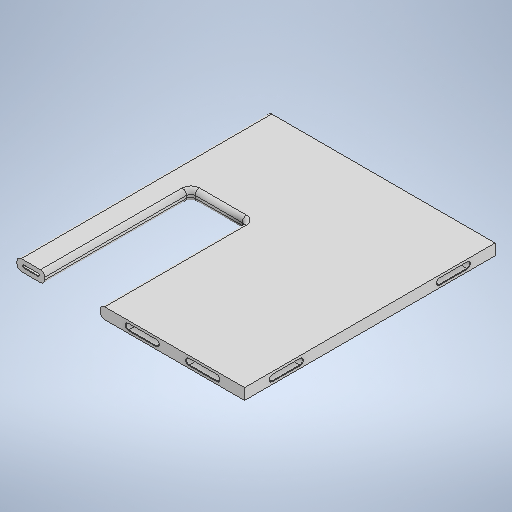
# Autodesk Inventor part: RightFlap4
Saved by Autodesk Inventor 2025.3 (Build 293356000, 356)
## iProperties
Created: 2025-11-19
Part Number: RightFlap4
Material: Generic
Document SubType Name: Modeling
Designer: User
Density: 1 g/cm^3
Appearance: Default
Author: User
Autodesk Inventor part; units mm, degrees
ref_plane "YZ Plane" through (0, 0, 0) normal (1, 0, 0) x (0, 1, 0)
ref_plane "XZ Plane" through (0, 0, 0) normal (0, 1, 0) x (-1, 0, 0)
ref_plane "XY Plane" through (0, 0, 0) normal (0, 0, 1) x (1, 0, 0)
sketch "Sketch1" plane through (0, 0, 0) normal (0, 1, 0) x (-1, 0, 0)
  line L0 (0, 0) -> (300, 0)
  line L1 (300, 0) -> (300, -420)
  line L2 (300, -420) -> (0, -420)
  line L3 (0, -420) -> (0, 0)
  line L4 (240, -150) -> (280, -150)
  line L5 (280, -150) -> (280, -270)
  line L6 (280, -270) -> (240, -270)
  line L7 (240, -270) -> (240, -150)
  line L8 (240, -150) -> (280, -270) construction
  line L9 (280, -150) -> (240, -270) construction
  dimension "d0" = 300
  dimension "d1" = 420
  dimension "d5" = 40
  dimension "d6" = 120
  constraints: 20 end point, 4 parallel, 2 horizontal, 2 perpendicular
  measures "d0" distance of L1.end L2.end
  measures "d1" distance of L0.end L1.end
  measures "d5" distance of L5.end L6.end
  measures "d6" distance of L4.end L5.end
extrude "Extrusion1" add sketch "Sketch1" along normal blind 8
sketch "Sketch2" plane through (0, 0, 0) normal (1, 0, 0) x (0, 0, -1)
  line L0 (150, 0) -> (270, 0) projected
  line L1 (210, 0) -> (210, 4)
  line L2 (420, 0) -> (420, 8) projected
  line L3 (0, 4.5) -> (420, 4.5)
  line L4 (420, 4.5) -> (420, 3.5)
  line L5 (420, 3.5) -> (0, 3.5)
  line L6 (0, 3.5) -> (0, 4.5)
  line L7 (0, 4.5) -> (420, 3.5) construction
  line L8 (420, 4.5) -> (0, 3.5) construction
  line L9 (0, 0) -> (0, 8) projected
  line L10 (420, 3.5) -> (0, 3.5)
  line L11 (0, 3.5) -> (0, 8)
  line L12 (0, 8) -> (420, 8)
  line L13 (420, 8) -> (420, 3.5)
  dimension "d7" = 4
  dimension "d8" = 1
  constraints: 22 end point, 4 parallel, 3 midpoint, 2 horizontal, 2 perpendicular, 1 point on line, 1 vertical
  measures "d7" distance of L1.start L1.end
  measures "d8" distance of L3.end L4.end
extrude "Extrusion2" cut sketch "Sketch2" against normal blind 40
fillet "Fillet1" radius 3.1 14 edges at (-300, 8, -210) (-300, 0, -210) (-280, 8, -210) (-260, 8, -270) (-240, 8, -210) (-280, 0, -210) (-260, 0, -270) (-280, 4, -270) (-240, 4, -270) (-240, 4, -150) (-260, 0, -150) (-260, 8, -150) (-280, 4, -150) (-240, 0, -210)
fillet "Fillet2" radius 2 11 edges at (-299.092, 7.092, 0) (-300, 4, 0) (-299.092, 0.908, 0) (-148.45, 0, 0) (-168.45, 8, 0) (-299.092, 7.092, -420) (-300, 4, -420) (-299.092, 0.908, -420) (-148.45, 0, -420) (-168.45, 8, -420) (0, 0, -210)
fillet "Fillet3" radius 0.3 8 edges at (-40, 7.4142, -419.4142) (-40, 4.75, -420) (-40, 7.4142, -0.5858) (-40, 4.75, 0) (-40, 8, -210) (-20, 3.5, -420) (0, 3.5, -210) (-20, 3.5, 0)
fillet "Fillet4" radius 2 6 edges at (-0.0879, 3.4121, -0.0879) (-0.5858, 0.5858, -0.5858) (0, 2.6, 0) (-0.0879, 3.4121, -419.9121) (-0.5858, 0.5858, -419.4142) (0, 2.6, -420)
mirror "Mirror1" about plane through (0, 0, 0) normal (1, 0, 0) remove original yes
sketch "Sketch3" plane through (2, 3.5, -0.3) normal (0, 1, 0) x (1, 0, 0)
  circle A0 centre (18, 14.7) radius 4.5
  line L0 (-1.7, 417.7) -> (-1.7, 1.7) construction
  line L1 (0, 0) -> (38, 0) projected
  circle A1 centre (18, 44.7) radius 4.5
  circle A2 centre (18, 74.7) radius 4.5
  line L2 (-2, 1.7) -> (-2, 417.7) projected
  line L3 (18, 74.7) -> (5.7787, 74.7)
  circle A3 centre (18, 134.7) radius 4.5
  circle A4 centre (18, 104.7) radius 4.5
  circle A5 centre (18, 74.7) radius 4.5
  line L4 (18, 134.7) -> (3.7207, 134.7)
  circle A6 centre (18, 194.7) radius 4.5
  line L5 (18, 194.7) -> (5.7787, 194.7)
  circle A7 centre (18, 164.7) radius 4.5
  circle A8 centre (18, 134.7) radius 4.5
  circle A9 centre (18, 254.7) radius 4.5
  line L6 (18, 254.7) -> (3.7207, 254.7)
  circle A10 centre (18, 224.7) radius 4.5
  circle A11 centre (18, 374.7) radius 4.5
  circle A12 centre (18, 344.7) radius 4.5
  circle A13 centre (18, 314.7) radius 4.5
  line L7 (18, 314.7) -> (5.7787, 314.7)
  circle A14 centre (18, 314.7) radius 4.5
  circle A15 centre (18, 284.7) radius 4.5
  circle A16 centre (18, 254.7) radius 4.5
  line L8 (18, 254.7) -> (3.7207, 254.7)
  circle A17 centre (18, 254.7) radius 4.5
  circle A18 centre (18, 224.7) radius 4.5
  circle A19 centre (18, 404.7) radius 4.5
  line L9 (0, 419.7) -> (38.3, 419.7) projected
  line L10 (38.3, -0.3) -> (0, -0.3) projected
  point P0 (-2, -0.3)
  dimension "d15" = 9
  dimension "d18" = 9
  dimension "d19" = 9
  dimension "d20" = 30
  dimension "d21" = 30
  dimension "d23" = 20
  dimension "d24" = 20
  dimension "d25" = 30
  dimension "d26" = 15
  dimension "d27" = 15
  constraints: 20 centre point, 14 symmetric about line, 12 end point, 2 horizontal, 16 other
  measures "d15" diameter of A0
  measures "d18" diameter of A1
  measures "d19" diameter of A2
  measures "d20" distance of A1.centre A0.centre
  measures "d21" distance of A1.centre L3.start
  measures "d23" distance from line of L2 A0.centre
  measures "d24" distance from line of L2 A19.centre
  measures "d25" distance of A19.centre A11.centre
  measures "d26" distance from line of L9 A19.centre
  measures "d27" distance from line of L10 A0.centre
extrude "Extrusion3" add sketch "Sketch3" along normal blind 2.5
fillet "Fillet5" radius 1 14 edges at (15.5, 6, -15) (15.5, 6, -45) (15.5, 6, -75) (15.5, 6, -105) (15.5, 6, -135) (15.5, 6, -165) (15.5, 6, -195) (15.5, 6, -225) (15.5, 6, -255) (15.5, 6, -285) (15.5, 6, -315) (15.5, 6, -345) (15.5, 6, -375) (15.5, 6, -405)
sketch "Sketch4" plane through (40.3, 8, -2) normal (0, 1, 0) x (1, 0, 0)
  line L0 (276.109, -16.9477) -> (96.109, -16.9477)
  line L1 (96.109, -16.9477) -> (96.109, 163.0523)
  line L2 (96.109, 163.0523) -> (276.109, 163.0523)
  line L3 (276.109, 163.0523) -> (276.109, -16.9477)
  line L4 (276.109, 163.0523) -> (96.109, 163.0523)
  line L5 (96.109, 163.0523) -> (96.109, 343.0523)
  line L6 (96.109, 343.0523) -> (276.109, 343.0523)
  line L7 (276.109, 343.0523) -> (276.109, 163.0523)
  line L8 (276.109, 343.0523) -> (96.109, 343.0523)
  line L9 (96.109, 343.0523) -> (96.109, 523.0523)
  line L10 (96.109, 523.0523) -> (276.109, 523.0523)
  line L11 (276.109, 523.0523) -> (276.109, 343.0523)
  line L12 (96.109, 163.0523) -> (-83.891, 163.0523)
  line L13 (-83.891, 163.0523) -> (-83.891, -16.9477)
  line L14 (-83.891, -16.9477) -> (96.109, -16.9477)
  line L15 (96.109, -16.9477) -> (96.109, 163.0523)
  line L16 (96.109, 163.0523) -> (-83.891, 163.0523)
  line L17 (-83.891, 163.0523) -> (-83.891, 343.0523)
  line L18 (-83.891, 343.0523) -> (96.109, 343.0523)
  line L19 (96.109, 343.0523) -> (96.109, 163.0523)
  line L20 (96.109, 343.0523) -> (-83.891, 343.0523)
  line L21 (-83.891, 343.0523) -> (-83.891, 523.0523)
  line L22 (-83.891, 523.0523) -> (96.109, 523.0523)
  line L23 (96.109, 523.0523) -> (96.109, 343.0523)
  point P0 (-40.3, -2)
  dimension "d31" = 180
  dimension "d32" = 180
  dimension "d33" = 180
  dimension "d34" = 180
  dimension "d35" = 180
  constraints: 48 end point, 12 parallel, 6 horizontal, 6 perpendicular, 5 point on line
  measures "d31" distance of L1.end L2.end
  measures "d32" distance of L0.end L1.end
  measures "d33" distance of L4.end L5.end
  measures "d34" distance of L8.end L9.end
  measures "d35" distance of L14.end L13.end
extrude "Extrusion4" cut sketch "Sketch4" against normal through all contours L0 L1 L2 L3 | L14 L13 L12 L1 | L12 L17 L18 L5 | L6 L9 L10 L11 | L18 L21 L22 L9
sketch "Sketch5" plane through (136.409, 8, -165.0523) normal (0, 0, 1) x (1, 0, 0)
  line L0 (148.5688, -4) -> (158.5688, -4) construction
  line L1 (148.5688, -4.75) -> (158.5688, -4.75)
  line L2 (158.5688, -3.25) -> (148.5688, -3.25)
  arc A0 (148.5688, -3.25) -> (148.5688, -4.75) centre (148.5688, -4) ccw
  arc A1 (158.5688, -4.75) -> (158.5688, -3.25) centre (158.5688, -4) ccw
  line L3 (20, -4) -> (40, -4) construction
  line L4 (20, -6) -> (40, -6)
  line L5 (40, -2) -> (20, -2)
  arc A2 (20, -2) -> (20, -6) centre (20, -4) ccw
  arc A3 (40, -6) -> (40, -2) centre (40, -4) ccw
  line L6 (0, 0) -> (0, -8) projected
  line L7 (63.591, -4) -> (83.591, -4) construction
  line L8 (63.591, -6) -> (83.591, -6)
  line L9 (83.591, -2) -> (63.591, -2)
  arc A4 (63.591, -2) -> (63.591, -6) centre (63.591, -4) ccw
  arc A5 (83.591, -6) -> (83.591, -2) centre (83.591, -4) ccw
  line L10 (103.591, -3.1) -> (103.591, -4.9) projected
  line L11 (160.491, 0) -> (0, 0) projected
  line L12 (86.9094, 0) -> (86.9094, -4)
  line L13 (0, -8) -> (160.491, -8) projected
  point P0 (-136.409, -8)
  point P1 (153.5688, -4)
  point P2 (30, -4)
  point P3 (73.591, -4)
  dimension "d38" = 5
  dimension "d39" = 1.5
  dimension "d40" = 10
  dimension "d41" = 4
  dimension "d42" = 30
  dimension "d43" = 10
  dimension "d44" = 4
  dimension "d45" = 30
  dimension "d46" = 4
  dimension "d47" = 4
  constraints: 26 end point, 12 point on circle, 12 tangent, 6 centre point, 3 horizontal, 3 midpoint, 3 parallel, 1 perpendicular, 1 point on line
  measures "d38" distance of point (153.569, -4) L0.end
  measures "d39" diameter of A1
  measures "d40" distance of point (30, -4) L3.end
  measures "d41" diameter of A3
  measures "d42" distance from line of L6 point (30, -4)
  measures "d43" distance of point (73.591, -4) L7.end
  measures "d44" diameter of A5
  measures "d45" distance from line of L10 point (73.591, -4)
  measures "d46" distance from line of L11 L7.start
  measures "d47" distance from line of L11 L3.end
extrude "Extrusion5" cut sketch "Sketch5" against normal blind 16
sketch "Sketch6" plane through (136.409, 8, -345.0523) normal (-1, 0, 0) x (0, 0, 1)
  line L0 (20, -4) -> (40, -4) construction
  line L1 (20, -6) -> (40, -6)
  line L2 (40, -2) -> (20, -2)
  arc A0 (20, -2) -> (20, -6) centre (20, -4) ccw
  arc A1 (40, -6) -> (40, -2) centre (40, -4) ccw
  line L3 (0, 0) -> (0, -8) projected
  line L4 (140.0415, -4) -> (160.0415, -4) construction
  line L5 (78.1523, -3.1) -> (180, -3.1) projected
  line L6 (140.0415, -6) -> (160.0415, -6)
  line L7 (160.0415, -2) -> (140.0415, -2)
  arc A2 (140.0415, -2) -> (140.0415, -6) centre (140.0415, -4) ccw
  arc A3 (160.0415, -6) -> (160.0415, -2) centre (160.0415, -4) ccw
  line L8 (150.0415, -4) -> (170.0415, -4) construction
  point P0 (345.0523, -8)
  point P1 (30, -4)
  point P2 (0, -4)
  dimension "d50" = 10
  dimension "d51" = 4
  dimension "d52" = 30
  dimension "d53" = 10
  dimension "d54" = 0
  dimension "d55" = 4
  constraints: 18 end point, 8 point on circle, 8 tangent, 4 centre point, 3 midpoint, 3 parallel, 2 horizontal, 1 collinear
  measures "d50" distance of point (30, -4) L0.end
  measures "d51" diameter of A1
  measures "d52" distance of point (0, -4) point (30, -4)
  measures "d53" distance of L8.start L4.end
  measures "d54" distance between parallel lines of L4 L8
  measures "d55" diameter of A3
extrude "Extrusion6" cut sketch "Sketch6" against normal blind 16
sketch "Sketch7" plane through (296.9, 8, -345.0523) normal (0, 0, -1) x (-1, 0, 0)
  line L0 (36.9, -4) -> (16.9, -4) construction
  line L1 (36.9, -2) -> (16.9, -2)
  line L2 (16.9, -6) -> (36.9, -6)
  arc A0 (36.9, -6) -> (36.9, -2) centre (36.9, -4) ccw
  arc A1 (16.9, -2) -> (16.9, -6) centre (16.9, -4) ccw
  line L3 (-3.1, -4.9) -> (-3.1, -3.1) projected
  line L4 (120.491, -4) -> (140.491, -4) construction
  line L5 (120.491, -6) -> (140.491, -6)
  line L6 (140.491, -2) -> (120.491, -2)
  arc A2 (120.491, -2) -> (120.491, -6) centre (120.491, -4) ccw
  arc A3 (140.491, -6) -> (140.491, -2) centre (140.491, -4) ccw
  line L7 (160.491, 0) -> (160.491, -8) projected
  point P0 (296.9, -8)
  point P1 (26.9, -4)
  point P2 (130.491, -4)
  dimension "d58" = 10
  dimension "d59" = 4
  dimension "d60" = 30
  dimension "d61" = 10
  dimension "d62" = 4
  dimension "d63" = 30
  constraints: 16 end point, 8 point on circle, 8 tangent, 4 centre point, 2 midpoint, 2 parallel, 2 point on line, 1 horizontal
  measures "d58" distance of point (26.9, -4) L0.end
  measures "d59" diameter of A1
  measures "d60" distance from line of L3 point (26.9, -4)
  measures "d61" distance of point (130.491, -4) L4.end
  measures "d62" diameter of A3
  measures "d63" distance from line of L7 point (130.491, -4)
extrude "Extrusion7" cut sketch "Sketch7" against normal blind 16
chamfer "Chamfer1" distance 0.3 angle 45 28 edges at (270, 6, -345.0523) (258, 4, -345.0523) (270, 2, -345.0523) (282, 4, -345.0523) (178.409, 4, -345.0523) (166.409, 6, -345.0523) (154.409, 4, -345.0523) (166.409, 2, -345.0523) (136.409, 4, -327.0523) (136.409, 6, -315.0523) (136.409, 4, -303.0523) (136.409, 2, -315.0523) (136.409, 4, -207.0108) (136.409, 6, -195.0108) (136.409, 4, -183.0108) (136.409, 2, -195.0108) (178.409, 4, -165.0523) (166.409, 2, -165.0523) (154.409, 4, -165.0523) (166.409, 6, -165.0523) (198, 4, -165.0523) (210, 6, -165.0523) (222, 4, -165.0523) (210, 2, -165.0523) (284.2278, 4, -165.0523) (289.9778, 4.75, -165.0523) (295.7278, 4, -165.0523) (289.9778, 3.25, -165.0523)
mirror "Mirror2" about plane through (136.409, 8, -345.0523) normal (-1, 0, 0) remove original yes
body "Solid1"
